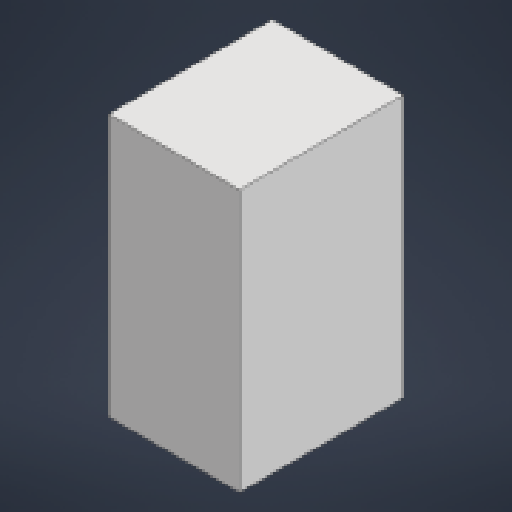
# Autodesk Inventor part: xy转接连杆
Saved by Autodesk Inventor 2025 (Build 290162000, 162)
## iProperties
Created: 2025-12-12
Part Number: xy转接连杆
Material: 常规
Document SubType Name: Modeling
Designer: HZD
Density: 1 g/cm^3
Appearance: 默认
Author: HZD
Autodesk Inventor part; units mm, degrees
ref_plane "YZ Plane" through (0, 0, 0) normal (1, 0, 0) x (0, 1, 0)
ref_plane "XZ Plane" through (0, 0, 0) normal (0, 1, 0) x (-1, 0, 0)
ref_plane "XY Plane" through (0, 0, 0) normal (0, 0, 1) x (1, 0, 0)
sketch "草图1" plane through (0, 0, 0) normal (0, 0, 1) x (1, 0, 0)
  line L0 (7.5, -20) -> (-7.5, -20)
  line L1 (-7.5, -20) -> (-7.5, 20)
  line L2 (-7.5, 20) -> (7.5, 20)
  line L3 (7.5, 20) -> (7.5, -20)
  line L4 (7.5, -20) -> (-7.5, 20) construction
  line L5 (-7.5, -20) -> (7.5, 20) construction
  point P0 (0, 0)
  dimension "d0" = 15
  dimension "d3" = 40
  constraints: 12 end point, 2 midpoint, 2 parallel, 1 horizontal, 1 perpendicular
  measures "d0" distance of L1.end L2.end
  measures "d3" distance of L0.end L1.end
extrude "拉伸1" add sketch "草图1" along normal blind 15
